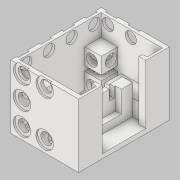
# Autodesk Inventor part: Bumper_back
Saved by Autodesk Inventor 2019.3 (Build 233278000, 278)
## iProperties
Created: 2019-02-26
Part Number: Bumper_back
Material: Generic
Document SubType Name: Modeling
Designer: Varga Daniel
Density: 1 g/cm^3
Appearance: White - P 1-1 C
Author: Varga Daniel
Autodesk Inventor part; units mm, degrees
ref_plane "YZ Plane" through (0, 0, 0) normal (1, 0, 0) x (0, 1, 0)
ref_plane "XZ Plane" through (0, 0, 0) normal (0, 1, 0) x (-1, 0, 0)
derived "Base_part.ipt"
sketch "Beam_sketch" plane through (0, 0, 0) normal (0, 1, 0) x (-1, 0, 0)
  line L0 (5, 0) -> (25, 0)
  line L1 (30, 5) -> (30, 25)
  line L2 (25, 30) -> (5, 30)
  line L3 (0, 25) -> (0, 5)
  line L4 (5, 29) -> (25, 29)
  line L5 (29, 25) -> (29, 5)
  line L6 (25, 1) -> (5, 1)
  line L7 (1, 5) -> (1, 25)
  circle A0 centre (5, 5) radius 2.5
  circle A1 centre (5, 5) radius 3.5
  arc A2 (25, 0) -> (30, 5) centre (25, 5) ccw
  arc A3 (30, 25) -> (25, 30) centre (25, 25) ccw
  arc A4 (5, 30) -> (0, 25) centre (5, 25) ccw
  arc A5 (0, 5) -> (5, 0) centre (5, 5) ccw
  arc A6 (1, 5) -> (5, 1) centre (5, 5) ccw
  arc A7 (5, 29) -> (1, 25) centre (5, 25) ccw
  arc A8 (29, 25) -> (25, 29) centre (25, 25) ccw
  arc A9 (25, 1) -> (29, 5) centre (25, 5) ccw
  line L8 (49.1041, 15) -> (-27.081, 15) construction
  line L9 (31.1478, 10) -> (-2.4877, 10) construction
  line L10 (-2.8604, 5) -> (35.495, 5) construction
  line L11 (5, -2.5736) -> (5, 36.7522) construction
  line L12 (15, -1.4978) -> (15, 34.8784) construction
  line L13 (1.5359, 5.5) -> (1, 5.5)
  line L14 (1.5359, 4.5) -> (1.0314, 4.5)
  line L15 (28.9686, 4.5) -> (8.4641, 4.5)
  line L16 (29, 5.5) -> (8.4641, 5.5)
  line L17 (4.5, 1.5359) -> (4.5, 1.0314)
  line L18 (5.5, 1.5359) -> (5.5, 1)
  line L19 (29, 10.5) -> (1, 10.5)
  line L20 (29, 9.5) -> (1, 9.5)
  line L21 (4.5, 28.9686) -> (4.5, 10.5)
  line L22 (4.5, 9.5) -> (4.5, 8.4641)
  line L23 (5.5, 29) -> (5.5, 10.5)
  line L24 (5.5, 9.5) -> (5.5, 8.4641)
  point P0 (0, 0)
  point P1 (30, 30)
  point P2 (0, 30)
  dimension "d4" = 7
  dimension "d3" = 5
  dimension "d5" = 1
  measures "d3" diameter of A0
  measures "d5" distance between parallel lines of L0 L6
sketch "Sketch1" plane through (0, 0, 0) normal (0, 1, 0) x (-1, 0, 0)
  line L0 (-15, -20) -> (15, -20)
  line L1 (15, -20) -> (15, 20)
  line L2 (15, 20) -> (-15, 20)
  line L3 (-15, 20) -> (-15, -20)
  line L4 (-15, -20) -> (15, 20) construction
  line L5 (15, -20) -> (-15, 20) construction
  line L6 (15, 0) -> (-15, 0) construction
  line L7 (0, 20) -> (0, -20) construction
  circle A0 centre (0, -15) radius 2.5
  circle A1 centre (0, -15) radius 3.85
  circle A2 centre (-10, -15) radius 2.5
  circle A3 centre (-10, -15) radius 3.85
  circle A4 centre (10, -15) radius 2.5
  circle A5 centre (10, -15) radius 3.85
  circle A6 centre (0, 15) radius 2.5
  circle A7 centre (0, 15) radius 3.85
  circle A8 centre (-10, 15) radius 2.5
  circle A9 centre (-10, 15) radius 3.85
  circle A10 centre (10, 15) radius 2.5
  circle A11 centre (10, 15) radius 3.85
  line L8 (13.1, 18) -> (13.1, -18)
  line L9 (13.1, -18) -> (-14, -18)
  line L10 (-14, -18) -> (-14, 18)
  line L11 (-14, 18) -> (13.1, 18)
  line L12 (-15, -9.6) -> (-14, -9.6)
  line L13 (13.1, 7.847) -> (-2.086, 7.847)
  line L14 (-2.086, 7.847) -> (-2.086, -7.847)
  line L15 (-2.086, -7.847) -> (13.1, -7.847)
  line L16 (13.1, -7.847) -> (13.1, 7.847)
  line L17 (-14, 9.6) -> (-15, 9.6)
  line L18 (-14, -11.15) -> (13.1, -11.15)
  line L19 (-14, 11.15) -> (13.1, 11.15)
  line L20 (-1.986, 7.747) -> (13, 7.747) construction
  line L21 (13, 7.747) -> (13, -7.747) construction
  line L22 (13, -7.747) -> (-1.986, -7.747) construction
  line L23 (-1.986, -7.747) -> (-1.986, 7.747) construction
  line L24 (-15, -14) -> (-14, -14)
  line L25 (-15, 14) -> (-14, 14)
  point P0 (13.1, -9.1)
  point P1 (13.1, 9.1)
  dimension "d0" = 40
  dimension "d1" = 30
  dimension "d6" = 5
  dimension "d7" = 7.7
  dimension "d10" = 10
  dimension "d17" = 10
  dimension "d22" = 30
  dimension "d42" = 10.4
  dimension "d43" = 10.4
  dimension "d50" = 0.1
  dimension "d51" = 0.1
  dimension "d52" = 0.1
  dimension "d53" = 0.1
  dimension "d57" = 30
  dimension "d59" = 1
  dimension "d60" = 6
  dimension "d61" = 6
  dimension "d79" = 2
  dimension "d80" = 2
  dimension "d119" = 6.85
  constraints: 52 end point, 15 point on line, 12 centre point, 10 parallel, 6 coincident, 6 horizontal, 6 symmetric about line, 4 midpoint, 3 vertical, 2 perpendicular, 2 tangent, 1 collinear, 18 other
  measures "d0" distance between parallel lines of L2 L0
  measures "d1" distance between parallel lines of L3 L1
  measures "d6" diameter of A0
  measures "d7" diameter of A1
  measures "d10" distance of A0.centre A2.centre
  measures "d17" distance of A0.centre A4.centre
  measures "d22" diameter of A0.centre L6
  measures "d42" distance between parallel lines of L17 L2
  measures "d43" distance between parallel lines of L12 L0
  measures "d50" distance between parallel lines of L23 L14
  measures "d51" distance between parallel lines of L13 L20
  measures "d52" distance between parallel lines of L15 L22
  measures "d53" distance between parallel lines of L21 L16
  measures "d57" distance of A2.centre A8.centre
  measures "d59" distance between parallel lines of L10 L3
  measures "d60" distance between parallel lines of L0 L24
  measures "d61" distance between parallel lines of L2 L25
  measures "d79" distance between parallel lines of L9 L0
  measures "d80" distance between parallel lines of L2 L11
  measures "d119" distance between parallel lines of L18 L9
extrude "Extrusion3" add sketch "Sketch1" against normal blind 2 contours L3 L24 L10 L9 A3 A1 A5 L8 A11 L11 A7 A9 L25 L2 L1 L0 | L3 L12 L10 L24 | L3 L17 L10 L12 | L10 L18 A3 L9 | L3 L25 L10 L17 | L10 L19 L8 L13 L14 L15 L18 | L18 A1 L9 A3 | L10 L11 A9 L19 | L18 A5 L9 A1 | A9 L11 A7 L19 | L18 L8 A5 | A7 L11 A11 L19 | A11 L8 L19 | L8 L9 A5 | L11 L8 A11 picked at (12.8847, -17.7742) picked at (12.8847, 17.7742)
extrude "Extrusion4" add sketch "Sketch1" against normal blind 1.2 from surface at 0 contours L9 A3 | A3 L9 | A1 L9 | A9 L11 | L9 A1 | A5 L8 L9 | A9 L11 | A7 L11 | A5 L8 | L9 A5 | A7 L11 | A11 L11 L8 | A11 L11 | L8 A11 picked at (12.9, -15) picked at (12.9, 15)
extrude "Extrusion8" add sketch "Sketch1" along normal blind 8.4 from surface at -1.2 contours L10 L18 A3 L9 | A3 L9 | L18 A1 L9 A3 | L10 L11 A9 L19 | L18 A5 L9 A1 | A1 L9 | A9 L11 | A9 L11 A7 L19 | L18 L8 A5 | A5 L8 L9 | A7 L11 | A7 L11 A11 L19 | A11 L11 L8 | A11 L8 L19 | L8 L9 A5 | L11 L8 A11 picked at (-10.1004, -17.8273) picked at (-0.1004, -17.8273) picked at (-10.1004, 17.8273) picked at (-0.1004, 17.8273)
sketch "Sketch4" plane through (0, 0, 0) normal (0, 1, 0) x (1, 0, 0)
  line L0 (0.986, 7.747) -> (-12, 7.747) construction
  line L1 (0.986, 7.747) -> (0.986, 8.947) construction
  line L2 (-12, 8.947) -> (0.986, 8.947) construction
  line L3 (-12, 7.747) -> (-12, 8.947) construction
  line L4 (-12, -7.747) -> (0.986, -7.747) construction
  line L5 (-12, -7.747) -> (-12, -8.947) construction
  line L6 (0.986, -8.947) -> (-12, -8.947) construction
  line L7 (0.986, -7.747) -> (0.986, -8.947) construction
  line L8 (2.086, 7.847) -> (-13.1, 7.847) projected
  line L9 (0.986, 8.947) -> (-12, 8.947)
  line L10 (-12, 8.947) -> (-12, 7.847)
  line L11 (-12, 7.847) -> (0.986, 7.847)
  line L12 (0.986, 7.847) -> (0.986, 8.947)
  line L13 (-13.1, -7.847) -> (2.086, -7.847) projected
  line L14 (0.986, -7.847) -> (-12, -7.847)
  line L15 (-12, -7.847) -> (-12, -8.947)
  line L16 (-12, -8.947) -> (0.986, -8.947)
  line L17 (0.986, -8.947) -> (0.986, -7.847)
  point P0 (0, 0)
  constraints: 16 end point, 4 collinear, 4 parallel, 4 point on line, 2 horizontal, 2 perpendicular
extrude "Extrusion9" add sketch "Sketch4" along normal blind 0.5
extrude "Extrusion10" add sketch "Sketch1" along normal blind 26 contours L3 L12 L10 L24 | L3 L25 L10 L17
ref_plane "Work Plane1" through (-14, 7.2, -18) normal (0, 1, 0) x (1, 0, 0)
sketch "Sketch6" plane through (-14, 7.2, -18) normal (0, 1, 0) x (1, 0, 0)
  line L0 (28, -8.4) -> (28, -6.85) projected
  line L1 (28, -4) -> (29, -4) projected
  line L2 (29, -4) -> (29, -8.4) projected
  line L3 (29, -8.4) -> (28, -8.4) projected
  line L4 (28, -29.15) -> (28, -27.6) projected
  line L5 (28, -27.6) -> (29, -27.6) projected
  line L6 (29, -27.6) -> (29, -32) projected
  line L7 (29, -32) -> (28, -32) projected
  line L8 (29, -8.9) -> (28, -8.9) projected
  line L9 (28, -8.4) -> (26, -8.4)
  line L10 (26, -8.4) -> (26, -6.85)
  line L11 (26, -6.85) -> (28, -6.85)
  line L12 (28, -6.85) -> (28, -8.4)
  line L13 (28, -27.6) -> (26, -27.6)
  line L14 (26, -27.6) -> (26, -29.15)
  line L15 (26, -29.15) -> (28, -29.15)
  line L16 (28, -29.15) -> (28, -27.6)
  line L17 (28, -6.85) -> (28, -4) projected
  line L18 (28, -6.85) -> (0.9, -6.85) projected
  line L19 (0.9, 0) -> (28, 0) projected
  line L20 (28, 0) -> (28, -4) projected
  line L21 (28, -32) -> (28, -29.15) projected
  line L22 (28, -32) -> (28, -36) projected
  line L23 (28, -36) -> (0.9, -36) projected
  line L24 (0.9, -29.15) -> (28, -29.15) projected
  circle A0 centre (4, -3) radius 2.5 projected
  circle A1 centre (24, -3) radius 2.5 projected
  circle A2 centre (14, -3) radius 2.5 projected
  circle A3 centre (24, -33) radius 2.5 projected
  circle A4 centre (4, -33) radius 2.5 projected
  circle A5 centre (14, -33) radius 2.5 projected
  line L25 (25.05, -21.7252) -> (25.05, -24.8892) construction
  line L26 (22.502, -24) -> (22.502, -23.25) construction
  line L27 (18.6, -6.85) -> (21.6, -6.85)
  line L28 (21.6, -6.85) -> (21.6, -8.4)
  line L29 (21.6, -8.4) -> (18.6, -8.4)
  line L30 (18.6, -8.4) -> (18.6, -6.85)
  line L31 (18.6, -29.15) -> (21.6, -29.15)
  line L32 (21.6, -29.15) -> (21.6, -27.6)
  line L33 (21.6, -27.6) -> (18.6, -27.6)
  line L34 (18.6, -27.6) -> (18.6, -29.15)
  line L35 (0.9, -6.85) -> (0.9, 0) projected
  line L36 (0.9, -36) -> (0.9, -29.15) projected
  point P0 (14, -18)
  dimension "d64" = 2
  dimension "d71" = 2
  dimension "d95" = 2.548
  dimension "d97" = 3
  dimension "d98" = 4.4
  constraints: 36 end point, 8 parallel, 6 collinear, 4 horizontal, 4 perpendicular, 2 point on line, 2 vertical, 4 other
  measures "d64" distance between parallel lines of L10 L0
  measures "d71" distance between parallel lines of L4 L14
  measures "d95" distance between parallel lines of L26 L25
  measures "d97" distance between parallel lines of L30 L28
  measures "d98" distance between parallel lines of L28 L10
extrude "Extrusion11" add sketch "Sketch6" along normal up to surface (18.8 mm away) contours L9 L10 L11 L0
extrude "Extrusion12" add sketch "Sketch6" against normal up to surface (7.2 mm away) contours L9 L10 L11 L0
extrude "Extrusion13" add sketch "Sketch6" along normal up to surface (18.8 mm away) contours L15 L14 L13 L4
extrude "Extrusion14" add sketch "Sketch6" against normal up to surface (7.2 mm away) contours L15 L14 L13 L4
sketch "Sketch7" plane through (0, 0, 0) normal (0, 1, 0) x (1, 0, 0)
  line L0 (7.6, 11.15) -> (5, 11.15)
  line L1 (5, 11.15) -> (5, -11.15)
  line L2 (5, -11.15) -> (7.6, -11.15)
  line L3 (7.6, -11.15) -> (7.6, 11.15)
  line L4 (14, -18) -> (-13.1, -18) construction
  line L5 (-13.1, -18) -> (-13.1, -11.15) construction
  line L6 (-13.1, -11.15) -> (12, -11.15) construction
  line L7 (12, -9.6) -> (15, -9.6) construction
  line L8 (15, 9.6) -> (15, -9.6) construction
  line L9 (15, 9.6) -> (12, 9.6) construction
  line L10 (12, 11.15) -> (-13.1, 11.15) construction
  line L11 (-13.1, 11.15) -> (-13.1, 18) construction
  line L12 (-13.1, 18) -> (14, 18) construction
  line L13 (14, 18) -> (14, 14) construction
  line L14 (14, 14) -> (15, 14) construction
  line L15 (15, 20) -> (15, 14) construction
  line L16 (-15, 20) -> (15, 20) construction
  line L17 (-15, -20) -> (-15, 20) construction
  line L18 (15, -20) -> (-15, -20) construction
  line L19 (15, -14) -> (15, -20) construction
  line L20 (15, -9.6) -> (15, -14) construction
  line L21 (14, -14) -> (14, -18) construction
  line L22 (15, -14) -> (14, -14) construction
  line L23 (15, 14) -> (15, 9.6) construction
  circle A0 centre (10, -15) radius 2.5 construction
  circle A1 centre (0, -15) radius 2.5 construction
  circle A2 centre (-10, -15) radius 2.5 construction
  line L24 (-13.1, 7.847) -> (-13.1, -7.847) construction
  line L25 (-13.1, -7.847) -> (-12, -7.847) construction
  line L26 (-12, -8.947) -> (-12, -7.847) construction
  line L27 (0.986, -8.947) -> (-12, -8.947) construction
  line L28 (0.986, -7.847) -> (0.986, -8.947) construction
  line L29 (0.986, -7.847) -> (2.086, -7.847) construction
  line L30 (2.086, -7.847) -> (2.086, 7.847) construction
  line L31 (2.086, 7.847) -> (0.986, 7.847) construction
  line L32 (0.986, 7.847) -> (-12, 7.847) construction
  line L33 (-12, 7.847) -> (-13.1, 7.847) construction
  line L34 (-12, -7.847) -> (0.986, -7.847) construction
  line L35 (0.986, 8.947) -> (0.986, 7.847) construction
  line L36 (-12, 8.947) -> (0.986, 8.947) construction
  line L37 (-12, 7.847) -> (-12, 8.947) construction
  circle A3 centre (-10, 15) radius 2.5 projected
  circle A4 centre (0, 15) radius 2.5 projected
  circle A5 centre (10, 15) radius 2.5 projected
  line L38 (12, 9.6) -> (12, 11.15) projected
  line L39 (12, -11.15) -> (12, -9.6) projected
  line L40 (12, 11.15) -> (-13.1, 11.15) construction
  line L41 (7.6, 11.15) -> (5, 11.15)
  line L42 (5, -11.15) -> (7.6, -11.15)
  line L43 (-13.1, -11.15) -> (12, -11.15) projected
  line L44 (5, -11.15) -> (3, -11.15)
  line L45 (3, -11.15) -> (3, -5.65)
  line L46 (3, -5.65) -> (5, -5.65)
  line L47 (5, -5.65) -> (5, -11.15)
  line L48 (5, 11.15) -> (3, 11.15)
  line L49 (3, 11.15) -> (3, 5.65)
  line L50 (3, 5.65) -> (5, 5.65)
  line L51 (5, 5.65) -> (5, 11.15)
  line L52 (5, 3.5) -> (3, 3.5)
  line L53 (3, 3.5) -> (3, -3.5)
  line L54 (3, -3.5) -> (5, -3.5)
  line L55 (5, -3.5) -> (5, 3.5)
  line L56 (8.502, 0) -> (5, 0) construction
  line L57 (7.6, 11.15) -> (7.6, 9.6) projected
  point P0 (0, 0)
  point P1 (4.002, -3.8)
  point P2 (7.6, 0)
  dimension "d86" = 5.5
  dimension "d87" = 2
  dimension "d88" = 5.5
  dimension "d89" = 7
  constraints: 38 end point, 8 parallel, 7 collinear, 4 horizontal, 4 perpendicular, 3 point on line, 2 midpoint, 1 vertical, 2 other
  measures "d86" distance between parallel lines of L10 L50
  measures "d87" distance between parallel lines of L53 L1
  measures "d88" distance between parallel lines of L46 L6
  measures "d89" distance between parallel lines of L52 L54
extrude "Extrusion15" add sketch "Sketch7" along normal blind 3.45 contours L3 L2 L1 L0
extrude "Extrusion16" add sketch "Sketch7" along normal blind 13 contours L1 L54 L53 L52
sketch "Sketch10" plane through (-13.1, 7.2, -18) normal (0, 1, 0) x (1, 0, 0)
  line L0 (20.7, -8.4) -> (17.7, -8.4) construction
  line L1 (20.7, -6.85) -> (20.7, -8.4) construction
  line L2 (20.7, -27.6) -> (17.7, -27.6) construction
  line L3 (20.7, -29.15) -> (20.7, -27.6) construction
  line L4 (0, -29.15) -> (25.1, -29.15) construction
  line L5 (25.1, -6.85) -> (0, -6.85) construction
  line L6 (18.1, -6.85) -> (18.1, -14.5) projected
  line L7 (20.7, -6.85) -> (18.1, -6.85)
  line L8 (18.1, -6.85) -> (18.1, -8.4)
  line L9 (18.1, -8.4) -> (20.7, -8.4)
  line L10 (20.7, -8.4) -> (20.7, -6.85)
  line L11 (20.7, -27.6) -> (18.1, -27.6)
  line L12 (18.1, -27.6) -> (18.1, -29.15)
  line L13 (18.1, -29.15) -> (20.7, -29.15)
  line L14 (20.7, -29.15) -> (20.7, -27.6)
  point P0 (13.1, -18)
  constraints: 16 end point, 3 parallel, 3 point on line, 2 horizontal, 2 perpendicular, 1 collinear
extrude "Extrusion17" add sketch "Sketch10" against normal up to surface (3.75 mm away)
sketch "Sketch11" plane through (14, 7.2, -18) normal (0, 0, -1) x (-1, 0, 0)
  circle A0 centre (4, -4.2) radius 2.5
  circle A1 centre (14, -4.2) radius 2.5
  circle A2 centre (24, -4.2) radius 2.5
  line L0 (29, -7.2) -> (29, -9.2) construction
  line L1 (-1, -7.2) -> (29, -7.2) construction
  line L2 (-1, -7.2) -> (-1, -9.2) construction
  line L3 (29, -9.2) -> (-1, -9.2) construction
  line L4 (29, -9.2) -> (-1, -9.2) construction
  point P0 (14, -7.2)
  dimension "d101" = 5
  dimension "d102" = 5
  dimension "d103" = 5
  dimension "d104" = 5
  dimension "d105" = 10
  dimension "d106" = 10
  dimension "d109" = 5
  dimension "d110" = 5
  dimension "d111" = 5
  constraints: 3 centre point
  measures "d101" diameter of A1
  measures "d102" diameter of A0
  measures "d103" diameter of A2
  measures "d104" distance from line of A0.centre L2
  measures "d105" distance of A1.centre A0.centre
  measures "d106" distance of A1.centre A2.centre
  measures "d109" distance from line of A2.centre L4
  measures "d110" distance from line of A1.centre L4
  measures "d111" distance from line of A0.centre L4
extrude "Extrusion19" cut sketch "Sketch11" against normal up to surface (6.85 mm away) contours A1 | A2
sketch "Sketch12" plane through (-13.1, 0, -11.15) normal (0, 0, 1) x (1, 0, 0)
  circle A0 centre (13.1, 3) radius 2.5 projected
  circle A1 centre (3.1, 3) radius 2.5 projected
  line L0 (18.1, 0) -> (18.1, 7.2) projected
  line L1 (18.1, 7.2) -> (0, 7.2) projected
  line L2 (0, 0) -> (0, 7.2) projected
  line L3 (18.1, 0) -> (0, 0) projected
  line L4 (16.6, 7.2) -> (0, 7.2)
  line L5 (0, 7.2) -> (0, 0)
  line L6 (0, 0) -> (16.6, 0)
  line L7 (16.6, 0) -> (16.6, 7.2)
  point P0 (13.1, 0)
  dimension "d116" = 1
  constraints: 8 end point, 2 parallel, 1 horizontal, 1 perpendicular, 1 point on line
  measures "d116" distance edge to line of A0 L7
extrude "Extrusion20" add sketch "Sketch12" along normal blind 0.35
sketch "Sketch13" plane through (-13.1, 7.2, 18) normal (0, 0, 1) x (1, 0, 0)
  circle A0 centre (3.1, -4.2) radius 2.5 projected
  circle A1 centre (13.1, -4.2) radius 2.5 projected
  line L0 (18.1, 0) -> (0, 0) projected
  line L1 (0, 0) -> (0, -7.2) projected
  line L2 (18.1, -7.2) -> (0, -7.2) projected
  line L3 (18.1, 0) -> (18.1, -7.2) projected
  point P0 (13.1, -7.2)
extrude "Extrusion21" cut sketch "Sketch13" against normal up to surface (6.85 mm away) contours A0 | A1
sketch "Sketch14" plane through (-13.1, 0, 11.15) normal (0, 0, -1) x (-1, 0, 0)
  circle A0 centre (-3.1, 3) radius 2.5 projected
  circle A1 centre (-13.1, 3) radius 2.5 projected
  line L0 (-18.1, 7.2) -> (0, 7.2) projected
  line L1 (0, 7.2) -> (0, 0) projected
  line L2 (-18.1, 0) -> (0, 0) projected
  line L3 (-18.1, 7.2) -> (-18.1, 0) projected
  point P0 (-13.1, 0)
extrude "Extrusion22" add sketch "Sketch14" along normal blind 0.35
sketch "Sketch15" plane through (-13.1, 7.2, -18) normal (0, 1, 0) x (1, 0, 0)
  line L0 (0, -28.8) -> (18.1, -28.8) projected
  line L1 (18.1, -28.8) -> (18.1, -21.5) projected
  line L2 (18.1, -21.5) -> (16.1, -21.5) projected
  line L3 (16.1, -21.5) -> (16.1, -14.5) projected
  line L4 (16.1, -14.5) -> (18.1, -14.5) projected
  line L5 (18.1, -14.5) -> (18.1, -7.2) projected
  line L6 (18.1, -7.2) -> (0, -7.2) projected
  line L7 (0, -7.2) -> (0, 0) projected
  line L8 (0, 0) -> (27.1, 0) projected
  line L9 (27.1, 0) -> (27.1, -4) projected
  line L10 (27.1, -4) -> (28.1, -4) projected
  line L11 (28.1, -4) -> (28.1, 2) projected
  line L12 (28.1, 2) -> (-1.9, 2) projected
  line L13 (-1.9, 2) -> (-1.9, -38) projected
  line L14 (-1.9, -38) -> (28.1, -38) projected
  line L15 (28.1, -38) -> (28.1, -32) projected
  line L16 (28.1, -32) -> (27.1, -32) projected
  line L17 (27.1, -32) -> (27.1, -36) projected
  line L18 (27.1, -36) -> (0, -36) projected
  line L19 (0, -36) -> (0, -28.8) projected
  line L20 (1.1, -10.153) -> (1.1, -9.053) projected
  line L21 (1.1, -9.053) -> (14.086, -9.053) projected
  line L22 (14.086, -9.053) -> (14.086, -10.153) projected
  line L23 (14.086, -10.153) -> (15.186, -10.153) projected
  line L24 (15.186, -10.153) -> (15.186, -25.847) projected
  line L25 (15.186, -25.847) -> (14.086, -25.847) projected
  line L26 (14.086, -25.847) -> (14.086, -26.947) projected
  line L27 (14.086, -26.947) -> (1.1, -26.947) projected
  line L28 (1.1, -26.947) -> (1.1, -25.847) projected
  line L29 (1.1, -25.847) -> (0, -25.847) projected
  line L30 (0, -25.847) -> (0, -10.153) projected
  line L31 (0, -10.153) -> (1.1, -10.153) projected
  circle A0 centre (3.1, -3) radius 2.5 projected
  circle A1 centre (23.1, -3) radius 2.5 projected
  circle A2 centre (13.1, -3) radius 2.5 projected
  line L32 (0, 0) -> (27.1, 0) projected
  line L33 (0, 0) -> (0, -7.2) projected
  line L34 (18.1, -7.2) -> (0, -7.2) projected
  line L35 (18.1, -7.2) -> (18.1, -8.4) projected
  line L36 (18.1, -8.4) -> (20.7, -8.4) projected
  line L37 (20.7, -8.4) -> (20.7, -6.85) projected
  line L38 (25.1, -6.85) -> (20.7, -6.85) projected
  line L39 (27.1, -6.85) -> (25.1, -6.85) projected
  line L40 (27.1, -4) -> (27.1, -6.85) projected
  line L41 (27.1, 0) -> (27.1, -4) projected
  line L42 (0, -36) -> (0, -28.8) projected
  line L43 (27.1, -36) -> (0, -36) projected
  line L44 (27.1, -32) -> (27.1, -36) projected
  line L45 (27.1, -29.15) -> (27.1, -32) projected
  line L46 (25.1, -29.15) -> (27.1, -29.15) projected
  line L47 (20.7, -29.15) -> (25.1, -29.15) projected
  line L48 (20.7, -29.15) -> (20.7, -27.6) projected
  line L49 (20.7, -27.6) -> (18.1, -27.6) projected
  line L50 (18.1, -27.6) -> (18.1, -28.8) projected
  line L51 (0, -28.8) -> (18.1, -28.8) projected
  circle A3 centre (13.1, -33) radius 2.5 projected
  circle A4 centre (3.1, -33) radius 2.5 projected
  circle A5 centre (23.1, -33) radius 2.5 projected
  line L52 (0, 0) -> (27.1, 0) projected
  line L53 (8.9, 0) -> (7.3, 0)
  line L54 (7.3, 0) -> (7.3, -7.2)
  line L55 (7.3, -7.2) -> (8.9, -7.2)
  line L56 (8.9, -7.2) -> (8.9, 0)
  line L57 (27.1, -36) -> (0, -36) projected
  line L58 (8.9, -28.8) -> (7.3, -28.8)
  line L59 (7.3, -28.8) -> (7.3, -36)
  line L60 (7.3, -36) -> (8.9, -36)
  line L61 (8.9, -36) -> (8.9, -28.8)
  line L62 (-1.9, 2) -> (-1.9, -38) projected
  point P0 (13.1, -18)
  dimension "d124" = 9.2
  dimension "d125" = 1.6
  dimension "d126" = 4.2
  dimension "d127" = 4.2
  constraints: 16 end point, 4 parallel, 4 point on line, 2 collinear, 2 horizontal, 2 perpendicular
  measures "d124" distance between parallel lines of L54 L62
  measures "d125" distance between parallel lines of L56 L54
  measures "d126" distance from line of L56 A2.centre
  measures "d127" distance from line of A0.centre L54
extrude "Extrusion23" cut sketch "Sketch15" against normal up to surface (7.2 mm away) contours L0 L61 L18 L59 | L6 L54 L8 L56
sketch "Sketch16" plane through (-13.1, 0, -18) normal (-1, 0, 0) x (0, 0, 1)
  line L0 (0, 7.2) -> (7.2, 7.2) construction
  line L1 (0, 7.2) -> (0, 0) construction
  line L2 (7.2, 0) -> (0, 0) construction
  line L3 (7.2, 7.2) -> (7.2, 0) construction
  line L4 (36, 7.2) -> (28.8, 7.2) construction
  line L5 (28.8, 0) -> (28.8, 7.2) construction
  line L6 (36, 0) -> (28.8, 0) construction
  line L7 (36, 7.2) -> (36, 0) construction
  line L8 (38, -2) -> (-2, -2) construction
  line L9 (38, 0) -> (38, -2) construction
  line L10 (-2, 0) -> (38, 0) construction
  line L11 (-2, 0) -> (-2, -2) construction
  line L12 (38, -2) -> (-2, -2) construction
  circle A0 centre (3, 3) radius 2.5
  circle A1 centre (33, 3) radius 2.5
  point P0 (18, 0)
  dimension "d130" = 5
  dimension "d131" = 5
  dimension "d132" = 5
  dimension "d133" = 5
  dimension "d134" = 5
  dimension "d135" = 5
  constraints: 2 centre point
  measures "d130" diameter of A0
  measures "d131" diameter of A1
  measures "d132" distance from line of A0.centre L11
  measures "d133" distance from line of A1.centre L9
  measures "d134" distance from line of A0.centre L8
  measures "d135" distance from line of A1.centre L8
extrude "Extrusion24" cut sketch "Sketch16" against normal up to surface (7.3 mm away)
sketch "Sketch17" plane through (0, 0, 0) normal (0, 1, 0) x (1, 0, 0)
  circle A0 centre (-10, -15) radius 2.5 projected
  line L0 (-5.8, 18) -> (-5.8, 10.8) projected
  line L1 (-5.8, 10.8) -> (-13.1, 10.8) projected
  line L2 (-13.1, 10.8) -> (-13.1, 18) projected
  line L3 (-13.1, 18) -> (-5.8, 18) projected
  line L4 (-5.8, -10.8) -> (-5.8, -18) projected
  line L5 (-5.8, -18) -> (-13.1, -18) projected
  line L6 (-13.1, -18) -> (-13.1, -10.8) projected
  line L7 (-13.1, -10.8) -> (-5.8, -10.8) projected
  line L8 (0.986, -7.847) -> (0.986, -8.947) projected
  line L9 (0.986, -8.947) -> (-12, -8.947) projected
  line L10 (-12, -8.947) -> (-12, -7.847) projected
  line L11 (-13.1, -7.847) -> (-12, -7.847) projected
  line L12 (-13.1, 7.847) -> (-13.1, -7.847) projected
  line L13 (-12, 7.847) -> (-13.1, 7.847) projected
  line L14 (-12, 7.847) -> (-12, 8.947) projected
  line L15 (-12, 8.947) -> (0.986, 8.947) projected
  line L16 (0.986, 8.947) -> (0.986, 7.847) projected
  line L17 (2.086, 7.847) -> (0.986, 7.847) projected
  line L18 (2.086, -7.847) -> (2.086, 7.847) projected
  line L19 (0.986, -7.847) -> (2.086, -7.847) projected
  line L20 (-12, -7.847) -> (0.986, -7.847) projected
  line L21 (0.986, 7.847) -> (-12, 7.847) projected
  circle A1 centre (-10, 15) radius 2.5 projected
  circle A2 centre (10, 15) radius 2.5 projected
  circle A3 centre (0, 15) radius 2.5 projected
  circle A4 centre (10, -15) radius 2.5 projected
  circle A5 centre (0, -15) radius 2.5 projected
  line L22 (-15, 20) -> (15, 20) projected
  line L23 (15, 20) -> (15, 14) projected
  line L24 (14, 14) -> (15, 14) projected
  line L25 (14, 18) -> (14, 14) projected
  line L26 (-4.2, 18) -> (14, 18) projected
  line L27 (-4.2, 10.8) -> (-4.2, 18) projected
  line L28 (5, 10.8) -> (-4.2, 10.8) projected
  line L29 (5, 3.5) -> (5, 10.8) projected
  line L30 (3, 3.5) -> (5, 3.5) projected
  line L31 (3, -3.5) -> (3, 3.5) projected
  line L32 (5, -3.5) -> (3, -3.5) projected
  line L33 (5, -10.8) -> (5, -3.5) projected
  line L34 (-4.2, -10.8) -> (5, -10.8) projected
  line L35 (-4.2, -18) -> (-4.2, -10.8) projected
  line L36 (14, -18) -> (-4.2, -18) projected
  line L37 (14, -14) -> (14, -18) projected
  line L38 (15, -14) -> (14, -14) projected
  line L39 (15, -9.6) -> (15, -14) projected
  line L40 (15, 9.6) -> (15, -9.6) projected
  line L41 (15, 14) -> (15, 9.6) projected
  line L42 (-15, -20) -> (-15, 20) projected
  line L43 (15, -20) -> (-15, -20) projected
  line L44 (15, -14) -> (15, -20) projected
  line L45 (12, -9.6) -> (15, -9.6) projected
  line L46 (12, -11.15) -> (12, -9.6) projected
  line L47 (7.6, -11.15) -> (12, -11.15) projected
  line L48 (7.6, 11.15) -> (7.6, -11.15) projected
  line L49 (12, 11.15) -> (7.6, 11.15) projected
  line L50 (12, 9.6) -> (12, 11.15) projected
  line L51 (15, 9.6) -> (12, 9.6) projected
  line L52 (14, 18) -> (-13.1, 18)
  line L53 (-13.1, 18) -> (-13.1, -18)
  line L54 (-13.1, -18) -> (14, -18)
  point P0 (0, 0)
  constraints: 6 end point, 2 perpendicular
extrude "Extrusion25" add sketch "Sketch17" along normal blind 26 contours L3 L2 L53 L12 L6 L5 L54 L36 L37 L38 L44 L43 L42 L22 L23 L24 L25 L26 L52
sketch "Sketch18" plane through (15, -2, -20) normal (0, 0, -1) x (-1, 0, 0)
  circle A0 centre (15, 5) radius 2.5 projected
  circle A1 centre (25, 5) radius 2.5 projected
  point P0 (15, 2)
extrude "Extrusion26" cut sketch "Sketch18" against normal up to next
sketch "Sketch19" plane through (15, -2, -20) normal (0, 0, -1) x (-1, 0, 0)
  circle A0 centre (15, 5) radius 2.5 projected
  circle A1 centre (25, 5) radius 2.5 projected
  line L0 (30, 0) -> (30, 28) projected
  line L1 (0, 28) -> (30, 28) projected
  line L2 (0, 28) -> (0, 0) projected
  line L3 (30, 0) -> (0, 0) projected
  arc A2 (23.2322, 3.2322) -> (26.7678, 3.2322) centre (25, 5) ccw projected
  circle A3 centre (25, 5) radius 3.85
  circle A4 centre (15, 5) radius 3.85
  point P0 (15, 2)
  dimension "d142" = 7.7
  dimension "d143" = 7.7
  constraints: 2 centre point, 2 coincident
  measures "d142" diameter of A3
  measures "d143" diameter of A4
extrude "Extrusion27" cut sketch "Sketch19" against normal blind 0.8 contours A3 | A4
sketch "Sketch20" plane through (-15, -2, 20) normal (0, 0, 1) x (1, 0, 0)
  circle A0 centre (15, 5) radius 2.5 projected
  circle A1 centre (5, 5) radius 2.5 projected
  point P0 (15, 2)
extrude "Extrusion28" cut sketch "Sketch20" against normal up to next
sketch "Sketch21" plane through (-15, -2, 20) normal (0, 0, 1) x (1, 0, 0)
  circle A0 centre (15, 5) radius 2.5 projected
  circle A1 centre (5, 5) radius 2.5 projected
  line L0 (30, 0) -> (30, 28) projected
  line L1 (0, 28) -> (30, 28) projected
  line L2 (0, 0) -> (0, 28) projected
  line L3 (30, 0) -> (0, 0) projected
  arc A2 (12.5, 5) -> (17.5, 5) centre (15, 5) ccw projected
  circle A3 centre (15, 5) radius 3.85
  circle A4 centre (5, 5) radius 3.85
  point P0 (15, 2)
  dimension "d148" = 7.7
  dimension "d149" = 7.7
  constraints: 2 centre point, 2 coincident
  measures "d148" diameter of A4
  measures "d149" diameter of A3
extrude "Extrusion29" cut sketch "Sketch21" against normal blind 0.8 contours A3 | A4
sketch "Sketch22" plane through (-15, -2, 20) normal (0, 0, 1) x (1, 0, 0)
  circle A0 centre (5, 25) radius 2.5
  circle A1 centre (15, 25) radius 2.5
  circle A2 centre (15, 5) radius 3.85 construction
  circle A3 centre (5, 5) radius 3.85 construction
  line L0 (30, 0) -> (30, 28) construction
  line L1 (0, 28) -> (30, 28) construction
  line L2 (0, 0) -> (0, 28) construction
  line L3 (30, 0) -> (0, 0) construction
  point P0 (15, 2)
  dimension "d152" = 5
  dimension "d153" = 5
  dimension "d154" = 25
  dimension "d155" = 25
  dimension "d156" = 5
  dimension "d157" = 10
  constraints: 2 centre point
  measures "d152" diameter of A1
  measures "d153" diameter of A0
  measures "d154" distance from line of A1.centre L3
  measures "d155" distance from line of A0.centre L3
  measures "d156" distance from line of A0.centre L2
  measures "d157" distance of A1.centre A0.centre
extrude "Extrusion30" cut sketch "Sketch22" against normal through all
sketch "Sketch23" plane through (-15, -2, 20) normal (0, 0, 1) x (1, 0, 0)
  circle A0 centre (5, 25) radius 2.5 construction
  circle A1 centre (15, 25) radius 2.5 construction
  circle A2 centre (15, 5) radius 3.85 construction
  circle A3 centre (5, 5) radius 3.85 construction
  line L0 (30, 0) -> (30, 28) construction
  line L1 (0, 28) -> (30, 28) projected
  line L2 (0, 0) -> (0, 28) construction
  line L3 (30, 0) -> (0, 0) construction
  arc A4 (17.413, 28) -> (12.587, 28) centre (15, 25) ccw
  circle A5 centre (5, 25) radius 3.85
  arc A6 (12.587, 28) -> (17.413, 28) centre (15, 25) ccw
  point P0 (15, 2)
  dimension "d160" = 7.7
  dimension "d161" = 7.7
  constraints: 4 point on circle, 3 centre point, 2 coincident, 2 point on line
  measures "d160" diameter of A4
  measures "d161" diameter of A5
extrude "Extrusion31" cut sketch "Sketch23" against normal blind 0.8
sketch "Sketch24" plane through (15, -2, -20) normal (0, 0, -1) x (-1, 0, 0)
  arc A0 (22.587, 28) -> (27.413, 28) centre (25, 25) ccw projected
  line L0 (30, 28) -> (27.413, 28) projected
  line L1 (30, 0) -> (30, 28) projected
  line L2 (0, 0) -> (30, 0) projected
  line L3 (0, 0) -> (0, 28) projected
  line L4 (12.587, 28) -> (0, 28) projected
  arc A1 (12.587, 28) -> (17.413, 28) centre (15, 25) ccw projected
  line L5 (22.587, 28) -> (17.413, 28) projected
  circle A2 centre (15, 5) radius 3.85 projected
  circle A3 centre (25, 5) radius 3.85 projected
  circle A4 centre (15, 25) radius 3.85
  circle A5 centre (25, 25) radius 3.85
  point P0 (15, 2)
  constraints: 2 centre point, 2 coincident, 2 concentric
extrude "Extrusion32" cut sketch "Sketch24" against normal blind 0.8 contours A5 A0 | A1 A4
sketch "Sketch26" plane through (-5.8, 0, -18) normal (0, 0, 1) x (1, 0, 0)
  circle A0 centre (-4.2, 23) radius 2.5 projected
  circle A1 centre (5.8, 23) radius 2.5 projected
  circle A2 centre (5.8, 3) radius 2.5 projected
  circle A3 centre (-4.2, 3) radius 2.5 projected
  line L0 (8.213, -1.2) -> (3.387, -1.2) projected
  line L1 (3.387, -1.2) -> (3.387, -2) projected
  line L2 (3.387, -2) -> (-1.787, -2) projected
  line L3 (-1.787, -2) -> (-1.787, -1.2) projected
  line L4 (-1.787, -1.2) -> (-6.613, -1.2) projected
  line L5 (-6.613, -1.2) -> (-6.613, -2) projected
  line L6 (-6.613, -2) -> (-9.2, -2) projected
  line L7 (-9.2, -2) -> (-9.2, 26) projected
  line L8 (-9.2, 26) -> (-7.3, 26) projected
  line L9 (-7.3, 26) -> (19.8, 26) projected
  line L10 (19.8, 26) -> (20.8, 26) projected
  line L11 (20.8, 26) -> (20.8, -2) projected
  line L12 (20.8, -2) -> (18.213, -2) projected
  line L13 (18.213, -2) -> (18.213, -1.2) projected
  line L14 (18.213, -1.2) -> (13.387, -1.2) projected
  line L15 (13.387, -1.2) -> (13.387, -2) projected
  line L16 (13.387, -2) -> (8.213, -2) projected
  line L17 (8.213, -2) -> (8.213, -1.2) projected
  line L18 (-7.3, 26) -> (-7.3, 7.2) projected
  line L19 (-7.3, 7.2) -> (0, 7.2) projected
  line L20 (0, 7.2) -> (0, 0) projected
  line L21 (0, 0) -> (1.6, 0) projected
  line L22 (1.6, 0) -> (1.6, 7.2) projected
  line L23 (1.6, 7.2) -> (19.8, 7.2) projected
  line L24 (19.8, 7.2) -> (19.8, 26) projected
  line L25 (-7.3, 16.6) -> (0, 16.6)
  line L26 (0, 16.6) -> (0, 9.4)
  line L27 (0, 9.4) -> (-7.3, 9.4)
  line L28 (-7.3, 9.4) -> (-7.3, 16.6)
  line L29 (0, 13) -> (-7.3, 13) construction
  point P0 (5.8, 0)
  dimension "d166" = 10
  constraints: 10 end point, 3 midpoint, 2 parallel, 1 collinear, 1 horizontal, 1 perpendicular
  measures "d166" distance from line of L29 A3.centre
extrude "Extrusion33" add sketch "Sketch26" along normal up to surface (7.2 mm away) contours L25 L26 L27 L18
sketch "Sketch27" plane through (15, -2, -20) normal (0, 0, -1) x (-1, 0, 0)
  arc A0 (12.587, 28) -> (17.413, 28) centre (15, 25) ccw projected
  line L0 (0, 28) -> (12.587, 28) projected
  line L1 (0, 28) -> (0, 0) projected
  line L2 (30, 0) -> (0, 0) projected
  line L3 (30, 0) -> (30, 28) projected
  line L4 (27.413, 28) -> (30, 28) projected
  arc A1 (22.587, 28) -> (27.413, 28) centre (25, 25) ccw projected
  line L5 (17.413, 28) -> (22.587, 28) projected
  circle A2 centre (15, 5) radius 3.85 projected
  circle A3 centre (25, 5) radius 3.85 projected
  circle A4 centre (25, 15) radius 2.5
  point P0 (15, 2)
  dimension "d169" = 5
  dimension "d170" = 5
  dimension "d171" = 15
  constraints: 1 centre point
  measures "d169" diameter of A4
  measures "d170" distance from line of A4.centre L3
  measures "d171" distance from line of A4.centre L2
sketch "Sketch28" plane through (-4.2, 0, 18) normal (0, 0, -1) x (-1, 0, 0)
  line L0 (1.6, 16.6) -> (1.6, 9.4) projected
  line L1 (8.9, 16.6) -> (1.6, 16.6) projected
  line L2 (8.9, 9.4) -> (8.9, 16.6) projected
  line L3 (1.6, 9.4) -> (8.9, 9.4) projected
  point P0 (-4.2, 0)
extrude "Extrusion34" add sketch "Sketch28" along normal up to surface (7.2 mm away)
extrude "Extrusion35" cut sketch "Sketch27" against normal through all contours A4
sketch "Sketch29" plane through (15, -2, -20) normal (0, 0, -1) x (-1, 0, 0)
  circle A0 centre (25, 15) radius 2.5 projected
  arc A1 (12.587, 28) -> (17.413, 28) centre (15, 25) ccw projected
  line L0 (0, 28) -> (12.587, 28) projected
  line L1 (0, 28) -> (0, 0) projected
  line L2 (30, 0) -> (0, 0) projected
  line L3 (30, 0) -> (30, 28) projected
  line L4 (27.413, 28) -> (30, 28) projected
  arc A2 (22.587, 28) -> (27.413, 28) centre (25, 25) ccw projected
  line L5 (17.413, 28) -> (22.587, 28) projected
  circle A3 centre (15, 5) radius 3.85 projected
  circle A4 centre (25, 5) radius 3.85 projected
  circle A5 centre (25, 15) radius 2.5 projected
  circle A6 centre (25, 15) radius 3.85
  point P0 (15, 2)
  dimension "d176" = 7.7
  constraints: 1 centre point, 1 coincident
  measures "d176" diameter of A6
extrude "Extrusion36" cut sketch "Sketch29" against normal blind 0.8 contours A6
sketch "Sketch30" plane through (-15, -2, 20) normal (0, 0, 1) x (1, 0, 0)
  circle A0 centre (5, 15) radius 3.85 projected
  point P0 (15, 2)
extrude "Extrusion37" cut sketch "Sketch30" against normal blind 0.8
sketch "Sketch31" plane through (-15, -2, -20) normal (-1, 0, 0) x (0, 0, 1)
  line L0 (40, 0) -> (40, 28) projected
  line L1 (0, 28) -> (40, 28) projected
  line L2 (0, 0) -> (0, 28) projected
  line L3 (40, 0) -> (0, 0) projected
  circle A0 centre (35, 25) radius 2.5
  circle A1 centre (35, 15) radius 2.5
  circle A2 centre (35, 5) radius 2.5
  circle A3 centre (25, 25) radius 2.5
  circle A4 centre (15, 25) radius 2.5
  circle A5 centre (5, 25) radius 2.5
  circle A6 centre (5, 15) radius 2.5
  circle A7 centre (5, 5) radius 2.5
  point P0 (20, 2)
  dimension "d181" = 5
  dimension "d183" = 5
  dimension "d186" = 10
  dimension "d193" = 10
  dimension "d200" = 10
  dimension "d207" = 5
  constraints: 8 centre point, 2 vertical, 1 horizontal, 14 other
  measures "d181" diameter of A0
  measures "d183" distance from line of A0.centre L0
  measures "d186" distance of A0.centre A1.centre
  measures "d193" distance of A0.centre A3.centre
  measures "d200" distance of A5.centre A6.centre
  measures "d207" distance from line of A2.centre L3
extrude "Extrusion38" cut sketch "Sketch31" against normal up to surface (1.9 mm away) contours A0 | A1 | A2 | A3 | A4 | A5 | A6 | A7
sketch "Sketch33" plane through (-15, -2, -20) normal (-1, 0, 0) x (0, 0, 1)
  circle A0 centre (5, 15) radius 2.5 projected
  circle A1 centre (5, 25) radius 2.5 projected
  circle A2 centre (25, 25) radius 2.5 projected
  circle A3 centre (35, 15) radius 2.5 projected
  circle A4 centre (35, 25) radius 2.5 projected
  circle A5 centre (15, 25) radius 2.5 projected
  line L0 (40, 0) -> (40, 28) projected
  line L1 (0, 28) -> (40, 28) projected
  line L2 (0, 0) -> (0, 28) projected
  line L3 (40, 0) -> (0, 0) projected
  point P0 (20, 2)
extrude "Extrusion39" cut sketch "Sketch33" against normal up to surface (9.2 mm away) contours A0 | A3
sketch "Sketch34" plane through (-15, -2, -20) normal (-1, 0, 0) x (0, 0, 1)
  circle A0 centre (5, 15) radius 2.5 projected
  circle A1 centre (5, 25) radius 2.5 projected
  circle A2 centre (25, 25) radius 2.5 projected
  circle A3 centre (35, 15) radius 2.5 projected
  circle A4 centre (35, 25) radius 2.5 projected
  circle A5 centre (15, 25) radius 2.5 projected
  line L0 (40, 0) -> (40, 28) projected
  line L1 (0, 28) -> (40, 28) projected
  line L2 (0, 0) -> (0, 28) projected
  line L3 (40, 0) -> (0, 0) projected
  circle A6 centre (35, 25) radius 3.85
  circle A7 centre (35, 15) radius 3.85
  circle A8 centre (35, 5) radius 3.85
  circle A9 centre (25, 25) radius 3.85
  circle A10 centre (15, 25) radius 3.85
  circle A11 centre (5, 25) radius 3.85
  circle A12 centre (5, 15) radius 3.85
  circle A13 centre (5, 5) radius 3.85
  dimension "d212" = 7.7
  dimension "d215" = 10
  dimension "d222" = 10
  dimension "d229" = 10
  constraints: 8 centre point, 2 vertical, 1 coincident, 1 horizontal, 14 other
  measures "d212" diameter of A6
  measures "d215" distance of A6.centre A7.centre
  measures "d222" distance of A6.centre A9.centre
  measures "d229" distance of A11.centre A12.centre
extrude "Extrusion40" cut sketch "Sketch34" against normal blind 0.8 contours A6 L1 | L1 A6 | A11 L1 | L1 A11 | A9 L1 | L1 A9 | A10 L1 | L1 A10 | A7 | A8 | A12 | A13
sketch "Sketch35" plane through (0, 3.45, 0) normal (0, 1, 0) x (1, 0, 0)
  line L0 (-15, 18.8236) -> (-15, 20) projected
  line L1 (-15, 20) -> (-13.8236, 20) projected
  line L2 (-13.8236, 20) -> (-13.8236, 19.2) projected
  line L3 (-13.8236, 19.2) -> (-12.4592, 19.2) projected
  line L4 (-12.4592, 19.2) -> (-12.4592, 17.4592) projected
  line L5 (-12.4592, 17.4592) -> (-14.2, 17.4592) projected
  line L6 (-13.1, 10.8) -> (-13.1, -10.8) projected
  line L7 (-13.1, -10.8) -> (-12.4592, -10.8) projected
  line L8 (-14.2, 12.5408) -> (-12.4592, 12.5408) projected
  line L9 (-12.4592, 12.5408) -> (-12.4592, 10.8) projected
  line L10 (-12.4592, 10.8) -> (-13.1, 10.8) projected
  line L11 (-6.1764, 20) -> (-3.8236, 20) projected
  line L12 (-3.8236, 20) -> (-3.8236, 19.2) projected
  line L13 (-3.8236, 19.2) -> (-2.4592, 19.2) projected
  line L14 (-2.4592, 19.2) -> (-2.4592, 15.45) projected
  arc A0 (-2.4592, 15.45) -> (-2.4592, 14.55) centre (0, 15) ccw projected
  line L15 (-2.4592, 14.55) -> (-2.4592, 10.8) projected
  line L16 (-2.4592, 10.8) -> (-4.2, 10.8) projected
  line L17 (-4.2, 10.8) -> (-4.2, 18) projected
  line L18 (-4.2, 18) -> (-5.8, 18) projected
  line L19 (-5.8, 18) -> (-5.8, 17.4592) projected
  line L20 (-7.5408, 19.2) -> (-6.1764, 19.2) projected
  line L21 (-6.1764, 19.2) -> (-6.1764, 20) projected
  line L22 (-13.8236, -19.2) -> (-13.8236, -20) projected
  line L23 (-13.8236, -20) -> (-15, -20) projected
  line L24 (-15, -20) -> (-15, -18.8236) projected
  line L25 (-14.2, -17.4592) -> (-12.4592, -17.4592) projected
  line L26 (-12.4592, -17.4592) -> (-12.4592, -19.2) projected
  line L27 (-12.4592, -19.2) -> (-13.8236, -19.2) projected
  line L28 (-5.8, -18) -> (-4.2, -18) projected
  line L29 (-4.2, -18) -> (-4.2, -10.8) projected
  line L30 (-4.2, -10.8) -> (-2.4592, -10.8) projected
  line L31 (-2.4592, -10.8) -> (-2.4592, -14.55) projected
  arc A1 (-2.4592, -14.55) -> (-2.4592, -15.45) centre (0, -15) ccw projected
  line L32 (-2.4592, -15.45) -> (-2.4592, -19.2) projected
  line L33 (-2.4592, -19.2) -> (-3.8236, -19.2) projected
  line L34 (-3.8236, -19.2) -> (-3.8236, -20) projected
  line L35 (-3.8236, -20) -> (-6.1764, -20) projected
  line L36 (-6.1764, -20) -> (-6.1764, -19.2) projected
  line L37 (-6.1764, -19.2) -> (-7.5408, -19.2) projected
  line L38 (-7.5408, -19.2) -> (-7.5408, -17.4592) projected
  line L39 (-7.5408, -17.4592) -> (-5.8, -17.4592) projected
  line L40 (-5.8, -17.4592) -> (-5.8, -18) projected
  line L41 (-7.5408, 12.5408) -> (-5.8, 12.5408) projected
  line L42 (-5.8, 12.5408) -> (-5.8, 10.8) projected
  line L43 (-5.8, 10.8) -> (-7.5408, 10.8) projected
  line L44 (-7.5408, -10.8) -> (-5.8, -10.8) projected
  line L45 (-5.8, -10.8) -> (-5.8, -12.5408) projected
  line L46 (7.6, -11.15) -> (12, -11.15) projected
  line L47 (12, -11.15) -> (12, -9.6) projected
  line L48 (12, -9.6) -> (15, -9.6) projected
  line L49 (15, -9.6) -> (15, -20) projected
  line L50 (15, -20) -> (3.8236, -20) projected
  line L51 (3.8236, -20) -> (3.8236, -19.2) projected
  line L52 (3.8236, -19.2) -> (2.4592, -19.2) projected
  line L53 (2.4592, -19.2) -> (2.4592, -15.45) projected
  arc A2 (2.4592, -15.45) -> (2.4592, -14.55) centre (0, -15) ccw projected
  line L54 (2.4592, -14.55) -> (2.4592, -10.8) projected
  line L55 (2.4592, -10.8) -> (5, -10.8) projected
  line L56 (5, -10.8) -> (5, -9.6) projected
  line L57 (5, -9.6) -> (7.6, -9.6) projected
  line L58 (7.6, 9.6) -> (7.6, -9.6) projected
  line L59 (7.6, 9.6) -> (5, 9.6) projected
  line L60 (5, 3.5) -> (5, 9.6) projected
  line L61 (3, 3.5) -> (5, 3.5) projected
  line L62 (3, -3.5) -> (3, 3.5) projected
  line L63 (5, -3.5) -> (3, -3.5) projected
  line L64 (5, -9.6) -> (5, -3.5) projected
  line L65 (7.6, -9.6) -> (7.6, -11.15) projected
  line L66 (7.6, 11.15) -> (7.6, 9.6) projected
  line L67 (12, 11.15) -> (7.6, 11.15) projected
  line L68 (12, 9.6) -> (12, 11.15) projected
  line L69 (15, 9.6) -> (12, 9.6) projected
  line L70 (15, 20) -> (15, 9.6) projected
  line L71 (3.8236, 20) -> (15, 20) projected
  line L72 (3.8236, 19.2) -> (3.8236, 20) projected
  line L73 (2.4592, 19.2) -> (3.8236, 19.2) projected
  line L74 (2.4592, 15.45) -> (2.4592, 19.2) projected
  arc A3 (2.4592, 14.55) -> (2.4592, 15.45) centre (0, 15) ccw projected
  line L75 (2.4592, 10.8) -> (2.4592, 14.55) projected
  line L76 (5, 10.8) -> (2.4592, 10.8) projected
  line L77 (5, 9.6) -> (5, 10.8) projected
  line L78 (5, 3.5) -> (5, -3.5) projected
  circle A4 centre (10, 15) radius 2.5 projected
  circle A5 centre (10, -15) radius 2.5 projected
  line L79 (5, 3.5) -> (5, 10.8) projected
  line L80 (7.6, 9.6) -> (5, 9.6)
  line L81 (5, 9.6) -> (5, 6.2)
  line L82 (5, 6.2) -> (7.6, 6.2)
  line L83 (7.6, 6.2) -> (7.6, 9.6)
  line L84 (5, -10.8) -> (5, -3.5) projected
  line L85 (7.6, -9.6) -> (5, -9.6)
  line L86 (5, -9.6) -> (5, -6.2)
  line L87 (5, -6.2) -> (7.6, -6.2)
  line L88 (7.6, -6.2) -> (7.6, -9.6)
  line L89 (-7.5408, 10.8) -> (-7.5408, 12.5408) projected
  line L90 (-7.5408, -12.5408) -> (-7.5408, -10.8) projected
  line L91 (-14.2, 18.8236) -> (-15, 18.8236) projected
  line L92 (-14.2, 17.4592) -> (-14.2, 18.8236) projected
  line L93 (-12.4592, -10.8) -> (-12.4592, -12.5408) projected
  line L94 (-12.4592, -12.5408) -> (-14.2, -12.5408) projected
  line L95 (-14.2, -12.5408) -> (-14.2, -11.1764) projected
  line L96 (-14.2, -11.1764) -> (-15, -11.1764) projected
  line L97 (-15, -11.1764) -> (-15, 11.1764) projected
  line L98 (-15, 11.1764) -> (-14.2, 11.1764) projected
  line L99 (-14.2, 11.1764) -> (-14.2, 12.5408) projected
  line L100 (-5.8, 17.4592) -> (-7.5408, 17.4592) projected
  line L101 (-7.5408, 17.4592) -> (-7.5408, 19.2) projected
  line L102 (-15, -18.8236) -> (-14.2, -18.8236) projected
  line L103 (-14.2, -18.8236) -> (-14.2, -17.4592) projected
  line L104 (-5.8, -12.5408) -> (-7.5408, -12.5408) projected
  point P0 (0, 0)
  dimension "d236" = 3.4
  dimension "d237" = 3.4
  constraints: 16 end point, 4 parallel, 2 horizontal, 2 perpendicular, 2 point on line
  measures "d236" distance between parallel lines of L82 L59
  measures "d237" distance between parallel lines of L87 L85
extrude "Extrusion41" add sketch "Sketch35" along normal up to surface (3.75 mm away) contours L57 L64 L87 L58 | L82 L60 L59 L58
sketch "Sketch36" plane through (0, 0, 0) normal (0, 1, 0) x (1, 0, 0)
  circle A0 centre (-10, -15) radius 2.5 projected
  line L0 (7.6, -11.15) -> (12, -11.15) projected
  line L1 (12, -11.15) -> (12, -9.6) projected
  line L2 (12, -9.6) -> (15, -9.6) projected
  line L3 (15, 9.6) -> (15, -9.6) projected
  line L4 (15, 20) -> (15, 9.6) projected
  line L5 (2.413, 20) -> (15, 20) projected
  line L6 (2.413, 19.2) -> (2.413, 20) projected
  line L7 (-2.413, 19.2) -> (2.413, 19.2) projected
  line L8 (-2.413, 20) -> (-2.413, 19.2) projected
  line L9 (-7.587, 20) -> (-2.413, 20) projected
  line L10 (-7.587, 19.2) -> (-7.587, 20) projected
  line L11 (-12.413, 19.2) -> (-7.587, 19.2) projected
  line L12 (-12.413, 20) -> (-12.413, 19.2) projected
  line L13 (-15, 20) -> (-12.413, 20) projected
  line L14 (-15, 17.413) -> (-15, 20) projected
  line L15 (-12.413, -20) -> (-15, -20) projected
  line L16 (-12.413, -19.2) -> (-12.413, -20) projected
  line L17 (-7.587, -19.2) -> (-12.413, -19.2) projected
  line L18 (-7.587, -20) -> (-7.587, -19.2) projected
  line L19 (-2.413, -20) -> (-7.587, -20) projected
  line L20 (-2.413, -19.2) -> (-2.413, -20) projected
  line L21 (2.413, -19.2) -> (-2.413, -19.2) projected
  line L22 (2.413, -20) -> (2.413, -19.2) projected
  line L23 (15, -20) -> (2.413, -20) projected
  line L24 (15, -9.6) -> (15, -20) projected
  line L25 (7.6, 11.15) -> (7.6, -11.15) projected
  line L26 (12, 11.15) -> (7.6, 11.15) projected
  line L27 (12, 9.6) -> (12, 11.15) projected
  line L28 (15, 9.6) -> (12, 9.6) projected
  line L29 (0.986, -7.847) -> (0.986, -8.947) projected
  line L30 (0.986, -8.947) -> (-12, -8.947) projected
  line L31 (-12, -8.947) -> (-12, -7.847) projected
  line L32 (-13.1, -7.847) -> (-12, -7.847) projected
  line L33 (-13.1, 7.847) -> (-13.1, -7.847) projected
  line L34 (-12, 7.847) -> (-13.1, 7.847) projected
  line L35 (-12, 7.847) -> (-12, 8.947) projected
  line L36 (-12, 8.947) -> (0.986, 8.947) projected
  line L37 (0.986, 8.947) -> (0.986, 7.847) projected
  line L38 (2.086, 7.847) -> (0.986, 7.847) projected
  line L39 (2.086, -7.847) -> (2.086, 7.847) projected
  line L40 (0.986, -7.847) -> (2.086, -7.847) projected
  line L41 (-12, -7.847) -> (0.986, -7.847) projected
  line L42 (-13.1, -7.847) -> (-13.1, -10.8) projected
  line L43 (-13.1, -10.8) -> (-5.8, -10.8) projected
  line L44 (-5.8, -10.8) -> (-5.8, -18) projected
  line L45 (-5.8, -18) -> (-4.2, -18) projected
  line L46 (-4.2, -18) -> (-4.2, -10.8) projected
  line L47 (-4.2, -10.8) -> (5, -10.8) projected
  line L48 (5, -10.8) -> (5, -3.5) projected
  line L49 (5, -3.5) -> (3, -3.5) projected
  line L50 (3, -3.5) -> (3, 3.5) projected
  line L51 (3, 3.5) -> (5, 3.5) projected
  line L52 (5, 3.5) -> (5, 10.8) projected
  line L53 (5, 10.8) -> (-4.2, 10.8) projected
  line L54 (-4.2, 10.8) -> (-4.2, 18) projected
  line L55 (-4.2, 18) -> (-5.8, 18) projected
  line L56 (-5.8, 18) -> (-5.8, 10.8) projected
  line L57 (-5.8, 10.8) -> (-13.1, 10.8) projected
  line L58 (-13.1, 10.8) -> (-13.1, 7.847) projected
  line L59 (0.986, 7.847) -> (-12, 7.847) projected
  circle A1 centre (-10, 15) radius 2.5 projected
  circle A2 centre (10, 15) radius 2.5 projected
  circle A3 centre (0, 15) radius 2.5 projected
  circle A4 centre (10, -15) radius 2.5 projected
  circle A5 centre (0, -15) radius 2.5 projected
  line L60 (-4.2, 18) -> (-4.2, 10.8) projected
  line L61 (5, 10.8) -> (-4.2, 10.8) projected
  line L62 (5, 10.8) -> (5, 6.2) projected
  line L63 (7.6, 6.2) -> (5, 6.2) projected
  line L64 (7.6, 6.2) -> (7.6, 11.15) projected
  line L65 (12, 11.15) -> (7.6, 11.15) projected
  line L66 (14, 11.15) -> (12, 11.15) projected
  line L67 (14, 18) -> (14, 11.15) projected
  line L68 (-4.2, 18) -> (14, 18) projected
  circle A6 centre (0, 15) radius 2.5 projected
  circle A7 centre (10, 15) radius 2.5 projected
  circle A8 centre (10, -15) radius 2.5 projected
  circle A9 centre (0, -15) radius 2.5 projected
  line L69 (-4.2, -10.8) -> (-4.2, -18) projected
  line L70 (14, -18) -> (-4.2, -18) projected
  line L71 (14, -11.15) -> (14, -18) projected
  line L72 (12, -11.15) -> (14, -11.15) projected
  line L73 (7.6, -11.15) -> (12, -11.15) projected
  line L74 (7.6, -6.2) -> (7.6, -11.15) projected
  line L75 (5, -6.2) -> (7.6, -6.2) projected
  line L76 (5, -6.2) -> (5, -10.8) projected
  line L77 (-4.2, -10.8) -> (5, -10.8) projected
  line L78 (5, 10.8) -> (3, 10.8)
  line L79 (3, 10.8) -> (3, 5.3)
  line L80 (3, 5.3) -> (5, 5.3)
  line L81 (5, 5.3) -> (5, 10.8)
  line L82 (5, -10.8) -> (3, -10.8)
  line L83 (3, -10.8) -> (3, -5.3)
  line L84 (3, -5.3) -> (5, -5.3)
  line L85 (5, -5.3) -> (5, -10.8)
  line L86 (-14.2, 17.413) -> (-15, 17.413) projected
  line L87 (-14.2, 12.587) -> (-14.2, 17.413) projected
  line L88 (-15, 12.587) -> (-14.2, 12.587) projected
  line L89 (-15, -12.587) -> (-15, 12.587) projected
  line L90 (-14.2, -12.587) -> (-15, -12.587) projected
  line L91 (-14.2, -17.413) -> (-14.2, -12.587) projected
  line L92 (-15, -17.413) -> (-14.2, -17.413) projected
  line L93 (-15, -20) -> (-15, -17.413) projected
  point P0 (0, 0)
  dimension "d240" = 5.5
  dimension "d241" = 5.5
  constraints: 16 end point, 4 parallel, 2 horizontal, 2 perpendicular, 1 collinear, 1 point on line
  measures "d240" distance between parallel lines of L78 L80
  measures "d241" distance between parallel lines of L84 L47
extrude "Extrusion42" add sketch "Sketch7" along normal up to surface (13 mm away) contours L1 L50 L49 L48 | L43 L45 L46 L1
sketch "Sketch37" plane through (12, 7.2, -11.15) normal (0, 1, 0) x (1, 0, 0)
  circle A0 centre (-2, 3.85) radius 2.5 projected
  circle A1 centre (-12, 3.85) radius 2.5 projected
  line L0 (-9, -0.35) -> (-9, 0) projected
  line L1 (-9, 0) -> (-7, 0) projected
  line L2 (-7, 0) -> (-7, -4.95) projected
  line L3 (-4.4, -4.95) -> (-7, -4.95) projected
  line L4 (-4.4, -4.95) -> (-4.4, 0) projected
  line L5 (0, 0) -> (-4.4, 0) projected
  line L6 (2, 0) -> (0, 0) projected
  line L7 (2, 6.85) -> (2, 0) projected
  line L8 (-16.2, 6.85) -> (2, 6.85) projected
  line L9 (-16.2, 6.85) -> (-16.2, -0.35) projected
  line L10 (-9, -0.35) -> (-16.2, -0.35) projected
  line L11 (-7, -17.35) -> (-7, -22.3) projected
  line L12 (-7, -22.3) -> (-9, -22.3) projected
  line L13 (-9, -22.3) -> (-9, -21.95) projected
  line L14 (-16.2, -21.95) -> (-9, -21.95) projected
  line L15 (-16.2, -21.95) -> (-16.2, -29.15) projected
  line L16 (2, -29.15) -> (-16.2, -29.15) projected
  line L17 (2, -22.3) -> (2, -29.15) projected
  line L18 (0, -22.3) -> (2, -22.3) projected
  line L19 (-4.4, -22.3) -> (0, -22.3) projected
  line L20 (-4.4, -17.35) -> (-4.4, -22.3) projected
  line L21 (-7, -17.35) -> (-4.4, -17.35) projected
  circle A2 centre (-12, -26.15) radius 2.5 projected
  circle A3 centre (-2, -26.15) radius 2.5 projected
  line L22 (-7, 0) -> (-4.4, 0)
  line L23 (-4.4, -22.3) -> (-7, -22.3)
  point P0 (-12, -11.15)
  constraints: 4 end point, 1 parallel
extrude "Extrusion43" add sketch "Sketch37" along normal up to surface (5.8 mm away) contours L22 L4 L3 L2 | L21 L20 L23 L11
sketch "Sketch38" plane through (0, 0, 0) normal (0, 1, 0) x (1, 0, 0)
  line L0 (3, -5.65) -> (5, -5.65) projected
  line L1 (5, -5.65) -> (5, -3.5) projected
  line L2 (5, -3.5) -> (3, -3.5) projected
  line L3 (3, -3.5) -> (3, 3.5) projected
  line L4 (3, 3.5) -> (5, 3.5) projected
  line L5 (5, 3.5) -> (5, 5.65) projected
  line L6 (5, 5.65) -> (3, 5.65) projected
  line L7 (3, 5.65) -> (3, 10.8) projected
  line L8 (3, 10.8) -> (-4.2, 10.8) projected
  line L9 (-4.2, 18) -> (-4.2, 10.8) projected
  line L10 (-4.2, 18) -> (-5.8, 18) projected
  line L11 (-5.8, 10.8) -> (-5.8, 18) projected
  line L12 (-5.8, 10.8) -> (-13.1, 10.8) projected
  line L13 (-13.1, 10.8) -> (-13.1, 7.847) projected
  line L14 (-13.1, 7.847) -> (-12, 7.847) projected
  line L15 (-12, 7.847) -> (-12, 8.947) projected
  line L16 (-12, 8.947) -> (0.986, 8.947) projected
  line L17 (0.986, 8.947) -> (0.986, 7.847) projected
  line L18 (0.986, 7.847) -> (2.086, 7.847) projected
  line L19 (2.086, 7.847) -> (2.086, -7.847) projected
  line L20 (2.086, -7.847) -> (0.986, -7.847) projected
  line L21 (0.986, -7.847) -> (0.986, -8.947) projected
  line L22 (0.986, -8.947) -> (-12, -8.947) projected
  line L23 (-12, -8.947) -> (-12, -7.847) projected
  line L24 (-12, -7.847) -> (-13.1, -7.847) projected
  line L25 (-13.1, -7.847) -> (-13.1, -10.8) projected
  line L26 (-13.1, -10.8) -> (-5.8, -10.8) projected
  line L27 (-5.8, -18) -> (-5.8, -10.8) projected
  line L28 (-5.8, -18) -> (-4.2, -18) projected
  line L29 (-4.2, -10.8) -> (-4.2, -18) projected
  line L30 (-4.2, -10.8) -> (3, -10.8) projected
  line L31 (3, -10.8) -> (3, -5.65) projected
  line L32 (5, 5.65) -> (3, 5.65) projected
  line L33 (3, 5.65) -> (3, 3.5)
  line L34 (3, -3.5) -> (3, 3.5) projected
  line L35 (3, -3.5) -> (3, -5.7143)
  line L36 (3, -10.8) -> (3, -5.65) projected
  point P0 (0, 0)
  constraints: 4 end point, 1 perpendicular, 1 point on line
extrude "Extrusion44" add sketch "Sketch38" along normal blind 8.5 contours L35 L2 L1 L0 | L33 L6 L5 L4
equation "\"d6\" = d3"
equation "\"d43\" = d42"
equation "\"d51\" = d50"
equation "\"d52\" = d50"
equation "\"d53\" = d50"
equation "\"d59\" = Wall_thickness"
equation "\"d61\" = d60"
equation "\"d80\" = d79"
equation "\"d38\" = d33 - 0.5 * Overall_height + 0.5 * Hole_height"
equation "\"d48\" = Hole_height"
equation "\"d71\" = d64"
equation "\"d88\" = d86"
equation "\"Wall_thickness\" = 1"
equation "\"d33\" = 2"
equation "\"Overall_height\" = 10"
equation "\"Hole_height\" = 8.4"
body "Solid2"
